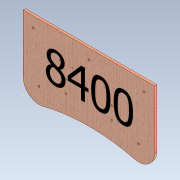
# Autodesk Inventor part: FTC Outside Panels
Saved by Autodesk Inventor 2020 (Build 240168000, 168)
## iProperties
Created: 2022-09-23
Part Number: FTC Outside Panels
Material: Wood (Oak)
Document SubType Name: Modeling
Designer: Jason
Density: 0.76 g/cm^3
Appearance: White Oak - Natural Medium Gloss
Mass: 371.39 g
Surface Area: 1832.51 cm^2
Volume: 488.671 cm^3
Author: Allan
Autodesk Inventor part; units mm, degrees
ref_plane "YZ Plane" through (0, 0, 0) normal (1, 0, 0) x (0, 1, 0)
ref_plane "XZ Plane" through (0, 0, 0) normal (0, 1, 0) x (-1, 0, 0)
ref_plane "XY Plane" through (0, 0, 0) normal (0, 0, 1) x (1, 0, 0)
sketch "Sketch1" plane through (0, 0, 0) normal (0, 0, 1) x (1, 0, 0)
  line L0 (40.3696, 0) -> (44.816, 0)
  line L1 (293.0054, 0) -> (287.9217, 0)
  arc A0 (0, 40.3696) -> (53.3921, 2.1581) centre (40.3696, 40.3696) ccw
  arc A1 (283.1915, 1.211) -> (333.375, 40.3696) centre (293.0054, 40.3696) ccw
  arc A2 (166.6875, 15.627) -> (44.816, 0) centre (166.3688, -464.9274) ccw
  arc A3 (287.9217, 0) -> (283.1915, 1.211) centre (166.3688, -464.9274) ccw
  arc A4 (53.3921, 2.1581) -> (44.816, 0) centre (166.3688, -464.9274) ccw
  arc A5 (287.9217, 0) -> (166.6875, 15.627) centre (166.3688, -464.9274) ccw
  line L2 (0, 40.3696) -> (0, 187.5234)
  line L3 (333.375, 187.5234) -> (333.375, 40.3696)
  line L4 (0, 187.5234) -> (333.375, 187.5234)
  point P0 (0, 0)
  point P1 (46.8129, 0.5175)
  dimension "d69" = 333.375
  constraints: 16 point on circle, 10 end point, 6 centre point, 1 perpendicular, 1 vertical
  measures "d69" distance between parallel lines of L3 L2
extrude "Extrusion1" add sketch "Sketch1" along normal blind 5.5563 contours A0 L2 L4 L3 A1 A5 A2
sketch "Sketch5" plane through (0, 0, 5.5563) normal (0, 0, 1) x (1, 0, 0)
  line L0 (53.8343, 140.6282) -> (283.9977, 140.6282) construction
  line L1 (283.9977, 140.6282) -> (283.9977, 59.079) construction
  line L2 (283.9977, 59.079) -> (53.8343, 59.079) construction
  line L3 (53.8343, 59.079) -> (53.8343, 140.6282) construction
  point P0 (0, 0)
  constraints: 2 other
sketch "Sketch6" plane through (0, 0, 5.5563) normal (0, 0, 1) x (1, 0, 0)
  line L0 (333.375, 187.5234) -> (0, 187.5234)
  line L1 (0, 187.5234) -> (0, 40.3696)
  circle A0 centre (26.0449, 161.4785) radius 2.4066
  line L2 (333.375, 40.3696) -> (333.375, 187.5234)
  circle A1 centre (307.3301, 161.4785) radius 2.4066
  circle A2 centre (166.6875, 161.4785) radius 2.4066
  arc A3 (283.1915, 1.211) -> (333.375, 40.3696) centre (293.0054, 40.3696) ccw
  circle A4 centre (293.0054, 40.3696) radius 2.4066
  arc A5 (0, 40.3696) -> (46.8129, 0.5175) centre (40.3696, 40.3696) ccw
  circle A6 centre (40.3696, 40.3696) radius 2.4066
  point P0 (0, 0)
  point P1 (0, 0)
  dimension "d70" = 333.375
  constraints: 7 centre point, 6 end point, 4 point on circle
  measures "d70" distance between parallel lines of L2 L1
extrude "Extrusion6" cut sketch "Sketch6" against normal up to surface (5.5563 mm away)
sketch "Sketch7" plane through (0, 0, 5.5563) normal (0, 0, 1) x (1, 0, 0)
  ellipse E0 centre (224.6285, 89.9888) end of major axis (224.6247, 91.9888) minor radius 2
  ellipse E1 centre (224.6285, 57.9868) end of major axis (224.6212, 59.9867) minor radius 2
  circle A0 centre (292.998, 40.3696) radius 2.9337
  line L0 (292.998, 40.3696) -> (224.6211, 40.3696)
  line L1 (224.6285, 40.3696) -> (224.6285, 57.9868)
  ellipse E2 centre (108.7466, 89.9867) end of major axis (108.7427, 91.9867) minor radius 2
  ellipse E3 centre (108.7466, 57.9868) end of major axis (108.7392, 59.9867) minor radius 2
  line L2 (108.7466, 40.3696) -> (108.7466, 57.9868)
  circle A1 centre (224.6594, 73.9878) radius 4.699
  circle A2 centre (108.7774, 73.9878) radius 4.699
  circle A3 centre (40.3696, 40.3696) radius 2.9337
  line L3 (40.3696, 40.3696) -> (108.7466, 40.3696)
  circle A4 centre (40.3696, 40.3696) radius 2.4066 projected
  circle A5 centre (293.0054, 40.3696) radius 2.4066 projected
  line L4 (40.3696, 40.3696) -> (293.0054, 40.3696)
  line L5 (224.6285, 89.9888) -> (224.6285, 57.9868)
  line L6 (108.7466, 89.9867) -> (108.7466, 57.9868)
  point P0 (0, 0)
  point P1 (0, 0)
  point P2 (166.6979, 70.2541)
  dimension "d59" = 17.6171
  dimension "d60" = 68.3769
  dimension "d61" = 17.6171
  dimension "d62" = 9.398
  dimension "d63" = 9.398
  dimension "d64" = 68.3769
  dimension "d71" = 252.6357
  dimension "d72" = 252.6284
  constraints: 14 end point, 4 centre point, 3 horizontal, 3 vertical, 1 coincident, 1 perpendicular, 8 other
  measures "d59" distance of L1.start L1.end
  measures "d60" distance of L0.end L0.start
  measures "d61" distance of L2.start L2.end
  measures "d62" diameter of A1
  measures "d63" diameter of A2
  measures "d64" distance of L3.end L3.start
  measures "d71" distance of L4.start L4.end
  measures "d72" distance of L0.start L3.start
extrude "Extrusion7" cut sketch "Sketch7" against normal through all contours E0 | E1 L5 L1 | L1 L5 E1 | E2 | E3 L6 L2 | L2 L6 E3
sketch "Sketch8" plane through (0, 0, 5.5563) normal (0, 0, 1) x (1, 0, 0)
  ellipse E0 centre (240.6029, 123.3584) end of major axis (240.6055, 122.0058) minor radius 1.3525
  ellipse E1 centre (208.6031, 123.2969) end of major axis (208.6057, 121.9443) minor radius 1.3525
  ellipse E2 centre (224.6285, 89.9888) end of major axis (224.6247, 91.9888) minor radius 2
  ellipse E3 centre (224.6285, 89.9888) end of major axis (224.6247, 91.9888) minor radius 2 projected
  ellipse E4 centre (124.721, 123.3562) end of major axis (124.7236, 122.0037) minor radius 1.3525
  ellipse E5 centre (92.7211, 123.2947) end of major axis (92.7237, 121.9422) minor radius 1.3525
  ellipse E6 centre (108.7466, 89.9867) end of major axis (108.7427, 91.9867) minor radius 2
  ellipse E7 centre (108.7466, 89.9867) end of major axis (108.7427, 91.9867) minor radius 2 projected
  point P0 (0, 0)
  constraints: 4 centre point, 6 other
extrude "Extrusion8" cut sketch "Sketch8" against normal through all contours E0 | E1 | E4 | E5
body "Solid1"
